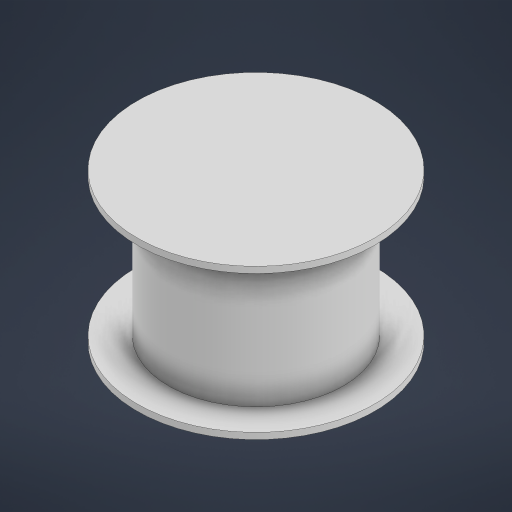
# Autodesk Inventor part: flywheels
Saved by Autodesk Inventor 2023 (Build 270158000, 158)
## iProperties
Created: 2022-05-21
Part Number: flywheels
Material: Generic
Document SubType Name: Modeling
Designer: jayso
Density: 1 g/cm^3
Appearance: Default
Author: jayso
Autodesk Inventor part; units mm, degrees
ref_plane "YZ Plane" through (0, 0, 0) normal (1, 0, 0) x (0, 1, 0)
ref_plane "XZ Plane" through (0, 0, 0) normal (0, 1, 0) x (-1, 0, 0)
ref_plane "XY Plane" through (0, 0, 0) normal (0, 0, 1) x (1, 0, 0)
sketch "Sketch1" plane through (0, 0, 0) normal (0, 1, 0) x (-1, 0, 0)
  circle A0 centre (0, -24) radius 19
  point P0 (0, 0)
  dimension "d1" = 38
  dimension "d3" = 24
  constraints: 1 centre point
  measures "d1" diameter of A0
  measures "d3" distance of point (0, 0) A0.centre
extrude "Extrusion1" add sketch "Sketch1" along normal blind 1
sketch "Sketch3" plane through (0, 1, -24) normal (0, 1, 0) x (1, 0, 0)
  circle A0 centre (0, 0) radius 14
  circle A1 centre (0, 0) radius 19
  circle A2 centre (0, 0) radius 19
  point P0 (0, -24)
  dimension "d7" = 28
  constraints: 3 centre point, 2 coincident
  measures "d7" diameter of A0
extrude "Extrusion3" add sketch "Sketch3" along normal blind 22 contours A0
sketch "Sketch5" plane through (0, 23, -24) normal (0, 1, 0) x (1, 0, 0)
  circle A0 centre (0, 0) radius 19
  point P0 (0, -24)
  constraints: 1 centre point
extrude "Extrusion5" add sketch "Sketch5" along normal blind 1
body "Solid1"
